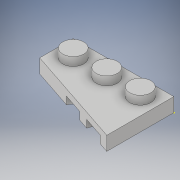
# Autodesk Inventor part: other diagonal piece
Saved by Autodesk Inventor 2017 (Build 210142000, 142)
## iProperties
Created: 2018-05-17
Part Number: other diagonal piece
Material: Generic
Document SubType Name: Modeling
Designer: 20000650
Density: 1 g/cm^3
Appearance: Default
Author: 20000650
Autodesk Inventor part; units mm, degrees
ref_plane "YZ Plane" through (0, 0, 0) normal (1, 0, 0) x (0, 1, 0)
ref_plane "XZ Plane" through (0, 0, 0) normal (0, 1, 0) x (-1, 0, 0)
ref_plane "XY Plane" through (0, 0, 0) normal (0, 0, 1) x (1, 0, 0)
sketch "Sketch1" plane through (0, 0, 0) normal (0, 1, 0) x (-1, 0, 0)
  line L0 (0, 0) -> (0, 15.5956)
  line L1 (0, 0) -> (23.3934, 0)
  line L2 (23.3934, 0) -> (23.3934, 7.7978)
  line L3 (23.3934, 7.7978) -> (0, 15.5956)
  dimension "d0" = 15.5956
  dimension "d1" = 23.3934
  dimension "d2" = 7.7978
  constraints: 8 end point, 2 vertical, 1 horizontal
  measures "d0" distance of L0.start L0.end
  measures "d1" distance of L0.start L1.end
  measures "d2" distance of L1.end L2.end
extrude "Extrusion1" add sketch "Sketch1" along normal blind 3.236
sketch "Sketch2" plane through (0, 3.236, 0) normal (0, 1, 0) x (1, 0, 0)
  line L0 (-23.3934, -7.7978) -> (0, -15.5956) projected
  line L1 (-23.3934, 0) -> (-23.3934, -7.7978)
  line L2 (0, 0) -> (-23.3934, 0) projected
  line L3 (-23.3934, 0) -> (-23.3934, -7.7978)
  circle A0 centre (-19.4945, -3.8989) radius 2.4498
  line L4 (-23.3934, 0) -> (-19.4945, 0) construction
  line L5 (-19.4945, 0) -> (-19.4945, -3.8989) construction
  line L6 (-19.4945, -3.8989) -> (-23.3934, -3.8989) construction
  line L7 (-23.3934, -3.8989) -> (-23.3934, 0) construction
  dimension "d7" = 4.8997
  dimension "d17" = 3.8989
  dimension "d18" = 3.8989
  constraints: 12 end point, 2 parallel, 1 centre point, 1 coincident, 1 horizontal, 1 perpendicular
  measures "d7" diameter of A0
  measures "d17" distance of L5.end L6.end
  measures "d18" distance of L4.end L5.end
extrude "Extrusion2" add sketch "Sketch2" along normal blind 1.9837
pattern_linear "Rectangular Pattern1" count 3 spacing 7.7978 along (1, 0, 0) of "Extrusion2"
sketch "Sketch3" plane through (0, 0, 0) normal (0, -1, 0) x (1, 0, 0)
  point P0 (0, 0)
shell "Shell1" thickness 1.4732 removed faces 1 at (-7.7978, 0, 7.7978)
sketch "Sketch4" plane through (-21.9202, 1.7628, 1.4732) normal (0, -1, 0) x (1, 0, 0)
  circle A0 centre (18.0213, 2.4257) radius 0.9766 construction
  circle A1 centre (10.2235, 2.4257) radius 0.9766 construction
  circle A2 centre (2.4257, 2.4257) radius 0.9766 construction
  line L0 (20.447, 12.0784) -> (20.447, 0) projected
  line L1 (0, 5.2628) -> (20.447, 12.0784) projected
  line L2 (0, 0) -> (0, 5.2628) construction
  line L3 (20.447, 0) -> (0, 0) construction
  circle A3 centre (18.0213, 2.4257) radius 2.4498 construction
  circle A4 centre (10.2235, 2.4257) radius 0.9766 construction
  circle A5 centre (10.2235, 2.4257) radius 2.4498 construction
  circle A6 centre (2.4257, 2.4257) radius 2.4498 construction
  line L4 (18.0213, 2.4257) -> (10.2235, 2.4257) construction
  line L5 (10.2235, 2.4257) -> (2.4257, 2.4257) construction
  line L6 (18.0213, 2.4257) -> (18.0213, 10.2235) construction
  line L7 (18.0213, 2.4257) -> (25.8191, 2.4257) construction
  line L8 (18.0213, 10.2235) -> (10.2235, 2.4257) construction
  circle A7 centre (14.1224, 6.3246) radius 3.064
  circle A8 centre (14.1224, 6.3246) radius 2.4498
  point P0 (21.9202, -1.4732)
  dimension "d14" = 7.7978
  dimension "d15" = 90
  dimension "d16" = 4.8997
  constraints: 10 end point, 2 centre point, 2 horizontal, 2 tangent, 1 coincident, 1 collinear, 1 midpoint, 1 perpendicular, 1 vertical
  measures "d14" distance of L4.start L6.end
  measures "d15" angle of L7 L6
  measures "d16" diameter of A8
extrude "Extrusion3" add sketch "Sketch4" along normal up to surface (1.7628 mm away)
pattern_linear "Rectangular Pattern2" count 2 spacing 7.7978 along (-1, 0, 0) of "Extrusion3"
sketch "Sketch5" plane through (-21.9202, 1.7628, 1.4732) normal (0, -1, 0) x (1, 0, 0)
  circle A0 centre (18.0213, 2.4257) radius 2.4498 construction
  line L0 (18.0213, 2.4257) -> (18.0213, 10.2235) construction
  line L1 (18.0213, 2.4257) -> (25.8191, 2.4257) construction
  circle A1 centre (18.0213, 10.2235) radius 2.4498 construction
  circle A2 centre (14.1224, 6.3246) radius 3.064 construction
  line L2 (15.6972, 9.4488) -> (13.6906, 15.4684) construction
  line L3 (13.6906, 15.4684) -> (19.2087, 14.4083) construction
  line L4 (19.2087, 14.4083) -> (20.3454, 10.9982) construction
  line L5 (21.9202, 14.1224) -> (7.2702, 9.2391) construction
  arc A3 (15.6972, 9.4488) -> (20.3454, 10.9982) centre (18.0213, 10.2235) ccw
  line L6 (20.3454, 10.9982) -> (19.2087, 14.4083)
  line L7 (15.6972, 9.4488) -> (13.6906, 15.4684)
  line L8 (13.6906, 15.4684) -> (19.2087, 14.4083)
  circle A4 centre (10.2235, 2.4257) radius 2.4498 construction
  line L9 (10.2235, 2.4257) -> (10.2235, 10.2235) construction
  line L10 (10.2235, 2.4257) -> (18.0213, 2.4257) construction
  circle A5 centre (10.2235, 10.2235) radius 2.4498 construction
  line L11 (13.4213, 8.3773) -> (11.5486, 13.9952) construction
  line L12 (11.5486, 13.9952) -> (1.2037, 10.5468) construction
  line L13 (1.2037, 10.5468) -> (2.2026, 7.5499) construction
  line L14 (3.8194, 8.0888) -> (-1.4732, 6.3246) construction
  line L15 (2.2026, 7.5499) -> (7.8994, 9.4488) construction
  arc A6 (13.1382, 9.2263) -> (11.9558, 8.4912) centre (14.1224, 6.3246) ccw construction
  arc A7 (13.1382, 9.2263) -> (11.9558, 8.4912) centre (14.1224, 6.3246) ccw
  arc A8 (7.8994, 9.4488) -> (11.9558, 8.4912) centre (10.2235, 10.2235) ccw
  line L16 (13.1382, 9.2263) -> (11.5486, 13.9952)
  line L17 (11.5486, 13.9952) -> (1.2037, 10.5468)
  line L18 (1.2037, 10.5468) -> (2.2026, 7.5499)
  line L19 (2.2026, 7.5499) -> (7.8994, 9.4488)
  point P0 (21.9202, -1.4732)
  dimension "d24" = 7.7978
  dimension "d25" = 90
  dimension "d28" = 7.7978
  dimension "d29" = 90
  constraints: 36 end point, 14 point on circle, 8 perpendicular, 7 tangent, 6 centre point, 4 collinear, 3 coincident, 2 concentric, 2 horizontal, 2 point on line, 2 vertical
  measures "d24" distance of L0.start L0.end
  measures "d25" angle of L1 L0
  measures "d28" distance of L9.start L9.end
  measures "d29" angle of L10 L9
extrude "Extrusion4" cut sketch "Sketch5" along normal up to surface (1.7628 mm away)
body "Solid1"
